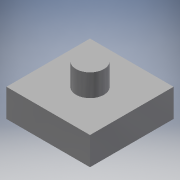
# Autodesk Inventor part: base
Saved by Autodesk Inventor 2017 (Build 210142000, 142)
## iProperties
Created: 2022-03-10
Part Number: base
Material: Stahl
Document SubType Name: Modeling
Designer: 10154704
Density: 7.85 g/cm^3
Appearance: Stahl
Author: 10154704
Autodesk Inventor part; units mm, degrees
ref_plane "YZ Plane" through (0, 0, 0) normal (1, 0, 0) x (0, 1, 0)
ref_plane "XZ Plane" through (0, 0, 0) normal (0, 1, 0) x (-1, 0, 0)
ref_plane "XY Plane" through (0, 0, 0) normal (0, 0, 1) x (1, 0, 0)
sketch "Skizze1" plane through (0, 0, 0) normal (0, 0, 1) x (1, 0, 0)
  line L0 (-15, 30) -> (15, 30)
  line L1 (15, 30) -> (15, 0)
  line L2 (15, 0) -> (-15, 0)
  line L3 (-15, 0) -> (-15, 30)
  point P0 (0, 0)
  dimension "d0" = 30
  dimension "d1" = 30
  dimension "d2" = 15
  constraints: 8 end point, 2 parallel, 1 horizontal, 1 midpoint, 1 perpendicular
  measures "d0" distance between parallel lines of L1 L3
  measures "d1" distance between parallel lines of L2 L0
  measures "d2" distance from line of L1 point (0, 0)
extrude "Extrusion1" add sketch "Skizze1" along normal blind 10
sketch "Skizze2" plane through (0, 0, 10) normal (0, 0, 1) x (1, 0, 0)
  line L0 (15, 0) -> (15, 30) projected
  line L1 (-15, 30) -> (-15, 0) projected
  line L2 (-15, 0) -> (15, 0) projected
  line L3 (15, 30) -> (-15, 30) projected
  circle A0 centre (0, 15) radius 5
  point P0 (0, 0)
  dimension "d5" = 30
  dimension "d6" = 30
  dimension "d7" = 15
  dimension "d8" = 15
  dimension "d9" = 10
  constraints: 1 centre point
  measures "d5" distance between parallel lines of L0 L1
  measures "d6" distance between parallel lines of L2 L3
  measures "d7" distance from line of L0 A0.centre
  measures "d8" distance from line of L2 A0.centre
  measures "d9" diameter of A0
extrude "Extrusion2" add sketch "Skizze2" along normal blind 8 contours A0
equation "\"d1\" = d0"
equation "\"d2\" = 0.5 * d0"
equation "\"d7\" = 0.5 * d5"
equation "\"d8\" = 0.5 * d6"
